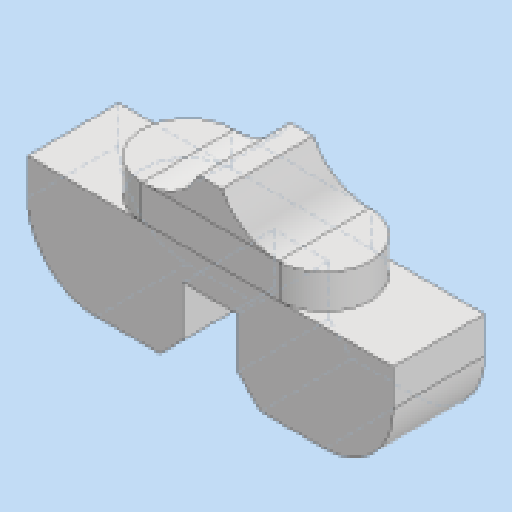
# Autodesk Inventor part: Sliding_switch
Saved by Autodesk Inventor 2024 (Build 280153000, 153)
## iProperties
Created: 2025-03-26
Part Number: Sliding_switch
Material: Generic
Document SubType Name: Modeling
Designer: XxPan
Density: 1 g/cm^3
Appearance: Default
Author: XxPan
Autodesk Inventor part; units mm, degrees
ref_plane "YZ Plane" through (0, 0, 0) normal (1, 0, 0) x (0, 1, 0)
ref_plane "XZ Plane" through (0, 0, 0) normal (0, 1, 0) x (-1, 0, 0)
ref_plane "XY Plane" through (0, 0, 0) normal (0, 0, 1) x (1, 0, 0)
sketch "Sketch1" plane through (0, 0, 0) normal (0, 1, 0) x (-1, 0, 0)
  line L0 (8, 2) -> (-8, 2)
  line L1 (-8, 2) -> (-8, -2)
  line L2 (-8, -2) -> (8, -2)
  line L3 (8, -2) -> (8, 2)
  line L4 (11.2, 0) -> (-11.2, 0) construction
  line L5 (0, -2.8) -> (0, 2.8) construction
  point P0 (0, 0)
  dimension "d0" = 16
  dimension "d1" = 4
  constraints: 8 end point, 2 parallel, 1 horizontal, 1 perpendicular, 2 other
  measures "d0" distance of L2.end L1.end
  measures "d1" distance of L0.end L1.end
extrude "Extrusion1" add sketch "Sketch1" against normal blind 4.6
sketch "Sketch2" plane through (-8, 0, 2) normal (0, 0, 1) x (1, 0, 0)
  line L0 (6.8, -1.4) -> (9.2, -1.4)
  line L1 (9.2, -1.4) -> (9.2, -4.6)
  line L2 (9.2, -4.6) -> (6.8, -4.6)
  line L3 (6.8, -4.6) -> (6.8, -1.4)
  line L4 (16, -4.6) -> (0, -4.6) projected
  point P0 (8, 0)
  point P1 (8, -4.6)
  point P2 (8, -4.6)
  dimension "d4" = 2.4
  dimension "d5" = 3.2
  constraints: 8 end point, 2 midpoint, 2 parallel, 1 coincident, 1 collinear, 1 horizontal, 1 perpendicular
  measures "d4" distance of L1.end L2.end
  measures "d5" distance of L0.end L1.end
extrude "Extrusion2" cut sketch "Sketch2" against normal through all
chamfer "Chamfer1" distance 1 angle 45 2 edges at (-1.2, -4.6, 0) (1.2, -4.6, 0)
fillet "Fillet1" radius 3 2 edges at (-8, -4.6, 0) (8, -4.6, 0)
sketch "Sketch3" plane through (0, 0, 0) normal (0, 1, 0) x (1, 0, 0)
  line L0 (-3, 0) -> (3, 0) construction
  line L1 (-3, -2.0001) -> (3, -2.0001)
  line L2 (3, 2.0001) -> (-3, 2.0001)
  arc A0 (-3, 2.0001) -> (-3, -2.0001) centre (-3, 0) ccw
  arc A1 (3, -2.0001) -> (3, 2.0001) centre (3, 0) ccw
  point P0 (0, 0)
  dimension "d12" = 3
  constraints: 8 end point, 4 point on circle, 4 tangent, 2 centre point, 1 horizontal, 1 midpoint, 1 parallel
  measures "d12" distance of point (0, 0) L0.end
extrude "Extrusion3" add sketch "Sketch3" along normal blind 1.5
sketch "Sketch4" plane through (0, 1.5, 0) normal (0, 1, 0) x (1, 0, 0)
  line L0 (-1.2, -2) -> (1.2, -2) projected
  line L1 (0.5, 2) -> (-0.5, 2)
  line L2 (-0.5, 2) -> (-0.5, -2)
  line L3 (-0.5, -2) -> (0.5, -2)
  line L4 (0.5, -2) -> (0.5, 2)
  line L5 (0.5, 2) -> (-0.5, -2) construction
  line L6 (-0.5, 2) -> (0.5, -2) construction
  point P0 (0, 0)
  dimension "d15" = 1
  constraints: 12 end point, 2 midpoint, 2 parallel, 1 horizontal, 1 perpendicular, 1 point on line
  measures "d15" distance of L3.end L2.end
extrude "Extrusion4" add sketch "Sketch4" along normal blind 1.5
fillet "Fillet2" radius 2.8 2 edges at (0.5, 1.5, 0) (-0.5, 1.5, 0)
body "Solid1"
